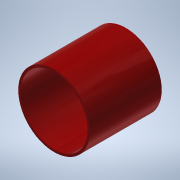
# Autodesk Inventor part: 筒
Saved by Autodesk Inventor 2020 (Build 240168000, 168)
## iProperties
Created: 2020-06-18
Part Number: 筒
Material: 一般
Document SubType Name: Modeling
Designer: jyajy
Density: 1 g/cm^3
Appearance: 既定
Author: jyajy
Autodesk Inventor part; units mm, degrees
ref_plane "YZ Plane" through (0, 0, 0) normal (1, 0, 0) x (0, 1, 0)
ref_plane "XZ Plane" through (0, 0, 0) normal (0, 1, 0) x (-1, 0, 0)
ref_plane "XY Plane" through (0, 0, 0) normal (0, 0, 1) x (1, 0, 0)
sketch "スケッチ1" plane through (0, 0, 0) normal (0, 0, 1) x (1, 0, 0)
  circle A0 centre (0, 0) radius 30
  circle A1 centre (0, 0) radius 28
  dimension "d0" = 60
  dimension "d21" = 2
  constraints: 2 centre point, 2 coincident
  measures "d0" diameter of A0
  measures "d21" radial gap between concentric circles of A0 A1
extrude "押し出し1" add sketch "スケッチ1" along normal blind 60
sketch "スケッチ6" plane through (0, 0, 0) normal (0, 0, -1) x (-1, 0, 0)
  circle A0 centre (0, 0) radius 28 projected
extrude "押し出し5" add sketch "スケッチ6" against normal blind 2
sketch "スケッチ7" plane through (0, 0, 0) normal (0, 0, -1) x (-1, 0, 0)
  line L0 (0, 0) -> (-30, 0)
  circle A0 centre (0, 0) radius 30 projected
  line L1 (0, 0) -> (0, 30)
  point P0 (-10, -15)
  point P1 (-10, 15)
  point P2 (10, -15)
  point P3 (10, 15)
  dimension "d24" = 20
  dimension "d25" = 30
  constraints: 4 end point, 3 symmetric about line, 2 point on circle, 1 perpendicular
  measures "d24" distance of point (10, -15) point (-10, -15)
  measures "d25" distance of point (-10, 15) point (-10, -15)
hole "穴2" at (10, -15, 0) at (10, 15, 0) at (-10, -15, 0) at (-10, 15, 0) direction (0, 0, 1) diameter 3.5 end through all
